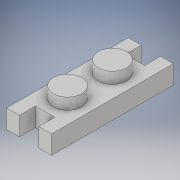
# Autodesk Inventor part: Weird circle things
Saved by Autodesk Inventor 2017 (Build 210142000, 142)
## iProperties
Created: 2018-05-11
Part Number: Weird circle things
Material: Generic
Document SubType Name: Modeling
Designer: Kyle
Density: 1 g/cm^3
Appearance: Default
Author: Kyle
Autodesk Inventor part; units mm, degrees
ref_plane "YZ Plane" through (0, 0, 0) normal (1, 0, 0) x (0, 1, 0)
ref_plane "XZ Plane" through (0, 0, 0) normal (0, 1, 0) x (-1, 0, 0)
ref_plane "XY Plane" through (0, 0, 0) normal (0, 0, 1) x (1, 0, 0)
sketch "Sketch1" plane through (0, 0, 0) normal (0, 1, 0) x (-1, 0, 0)
  line L0 (0, 0) -> (7.7978, 0) construction
  line L1 (7.7978, 0) -> (7.7978, -21.1531) construction
  line L2 (7.7978, -21.1531) -> (0, -21.1531) construction
  line L3 (0, -21.1531) -> (0, 0) construction
  line L4 (7.7978, -10.5766) -> (7.7978, -2.7788) construction
  line L5 (7.7978, -2.7788) -> (0, -2.7788) construction
  line L6 (0, -2.7788) -> (0, -18.3744) construction
  line L7 (0, -18.3744) -> (7.7978, -18.3744) construction
  line L8 (7.7978, -18.3744) -> (7.7978, -2.7788) construction
  line L9 (7.7978, 0) -> (5.5905, 0) construction
  line L10 (5.5905, 0) -> (5.5905, -2.7788) construction
  line L11 (5.5905, -2.7788) -> (7.7978, -2.7788) construction
  line L12 (7.7978, -2.7788) -> (7.7978, 0) construction
  line L13 (7.7978, -10.5766) -> (0, -10.5766) construction
  line L14 (5.5905, -21.1531) -> (5.5905, -18.3744) construction
  line L15 (3.8989, 0) -> (3.8989, -21.1531) construction
  line L16 (2.2073, 0) -> (2.2073, -2.7788) construction
  line L17 (2.2073, -21.1531) -> (2.2073, -18.3744) construction
  line L18 (7.7978, 0) -> (7.7978, -21.1531)
  line L19 (7.7978, -21.1531) -> (5.5905, -21.1531)
  line L20 (5.5905, -21.1531) -> (5.5905, -18.3744)
  line L21 (5.5905, -18.3744) -> (2.2073, -18.3744)
  line L22 (2.2073, -18.3744) -> (2.2073, -21.1531)
  line L23 (2.2073, -21.1531) -> (0, -21.1531)
  line L24 (0, -21.1531) -> (0, 0)
  line L25 (0, 0) -> (2.2073, 0)
  line L26 (2.2073, 0) -> (2.2073, -2.7788)
  line L27 (2.2073, -2.7788) -> (5.5905, -2.7788)
  line L28 (5.5905, -2.7788) -> (5.5905, 0)
  line L29 (5.5905, 0) -> (7.7978, 0)
  dimension "d0" = 7.7978
  dimension "d1" = 21.1531
  dimension "d2" = 7.7978
  dimension "d3" = 7.7978
  dimension "d4" = 15.5956
  dimension "d5" = 2.2073
  constraints: 60 end point, 6 collinear, 6 parallel, 6 symmetric about line, 5 perpendicular, 4 midpoint, 3 horizontal, 2 point on line
  measures "d0" distance of L1.end L2.end
  measures "d1" distance of L0.end L1.end
  measures "d2" distance of L4.start L4.end
  measures "d3" distance of L7.end L6.end
  measures "d4" distance of L6.end L5.end
  measures "d5" distance of L11.end L10.end
extrude "Extrusion1" add sketch "Sketch1" along normal blind 3.236
sketch "Sketch2" plane through (0, 3.236, 0) normal (0, 1, 0) x (1, 0, 0)
  line L0 (0, 0) -> (0, 21.1531) construction
  line L1 (0, 10.5766) -> (-7.7978, 10.5766) construction
  line L2 (-7.7978, 21.1531) -> (-7.7978, 0) construction
  line L3 (0, 10.5766) -> (-3.8989, 10.5766) construction
  line L4 (-3.8989, 10.5766) -> (-3.8989, 6.6777) construction
  line L5 (-3.8989, 6.6777) -> (0, 6.6777) construction
  line L6 (0, 6.6777) -> (0, 10.5766) construction
  circle A0 centre (-3.8989, 6.6777) radius 2.4498
  dimension "d8" = 3.8989
  dimension "d9" = 3.8989
  dimension "d10" = 4.8997
  constraints: 10 end point, 2 midpoint, 2 parallel, 1 centre point, 1 coincident, 1 horizontal, 1 perpendicular
  measures "d8" distance of L5.end L4.end
  measures "d9" distance of L4.end L3.end
  measures "d10" diameter of A0
extrude "Extrusion2" add sketch "Sketch2" along normal blind 1.9837
pattern_linear "Rectangular Pattern1" count 2 spacing 7.7978 along (0, 0, -1) of "Extrusion2"
shell "Shell1" thickness 1.4732 removed faces 1 at (-3.335, 0, -7.9773)
sketch "Sketch3" plane through (-6.3246, 1.7628, -16.9012) normal (0, -1, 0) x (1, 0, 0)
  circle A0 centre (2.4257, 10.2235) radius 2.4498 construction
  circle A1 centre (2.4257, 2.4257) radius 2.4498 construction
  line L0 (2.4257, 10.2235) -> (2.4257, 2.4257) construction
  circle A2 centre (2.4257, 6.3246) radius 1.4491
  point P0 (6.3246, 16.9012)
  constraints: 2 end point, 1 centre point, 1 midpoint, 1 vertical
extrude "Extrusion3" add sketch "Sketch3" along normal up to surface (1.7628 mm away)
body "Solid1"
